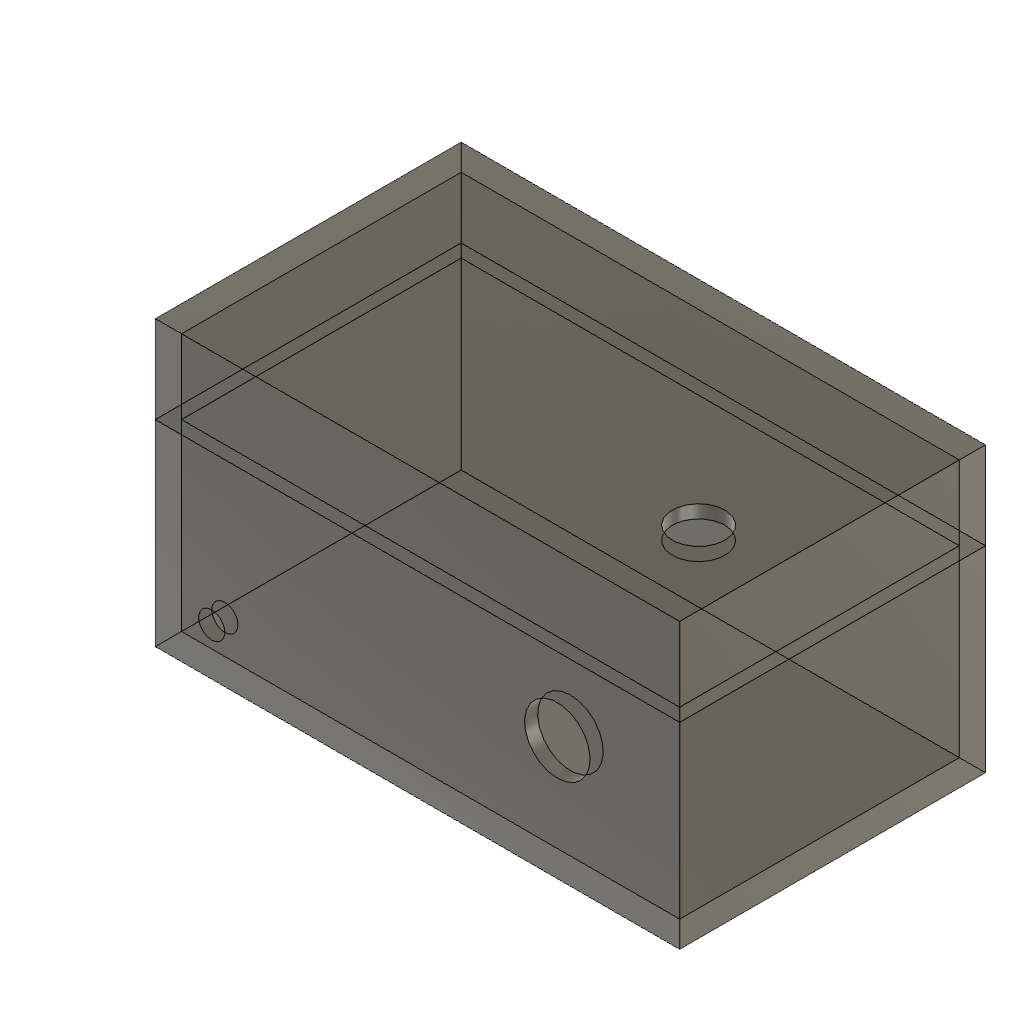
12345 (Autodesk Fusion 360 design; units mm, degrees)
Autodesk Fusion 360 part; units mm, degrees
sketch "Sketch1" plane through (0, 0, 0) normal (0, 0, 1) x (1, 0, 0)
  line L0 (0, 0) -> (120, 0)
  line L1 (120, 0) -> (120, 70)
  line L2 (120, 70) -> (0, 70)
  line L3 (0, 70) -> (0, 0)
  dimension "d1" = 70
  dimension "d2" = 120
  constraint horizontal L0
  constraint vertical L1
  constraint horizontal L2
  constraint vertical L3
  constraint coincident L0.start L3.end
  measures "d1" distance of L0.start L2.end
  measures "d2" distance of L0.start L0.end
extrude "Extrude1" add sketch "Sketch1" along normal blind 65 makes body 1
shell "Shell1" thickness 3 removed faces 0 bodies 1
ref_plane "WorkPlane1" through (0, 0, 45) normal (0, 0, 1) x (1, 0, 0)
split "Split1" by plane through (0, 0, 45) normal (0, 0, 1) bodies 1 makes body 2 at (40, 46.6667, 65)
hole "Hole1" at (12.922, 3, 10.7655) direction (0, -1, 0) diameter 6 depth 20 tip angle 118 bodies 1
hole "Hole2" at (92.0095, 3, 27.4311) direction (0, -1, 0) diameter 15 depth 20 tip angle 118 bodies 1
hole "Hole3" at (103.0871, 21.2472, 62) direction (0, 0, 1) diameter 12 depth 20 tip angle 118 bodies 2
